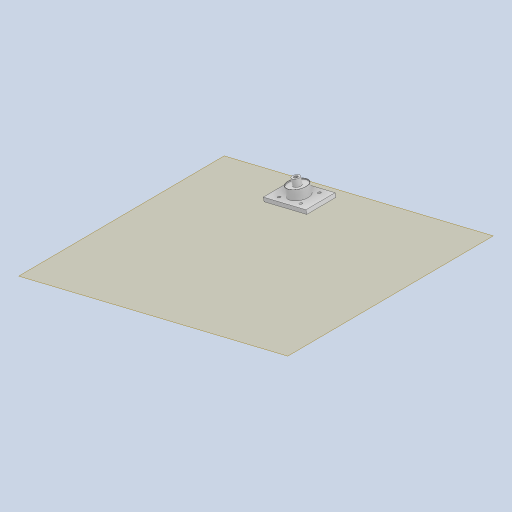
# Autodesk Inventor part: ступица
Saved by Autodesk Inventor 2024.2 (Build 282272000, 272)
## iProperties
Created: 2025-12-13
Part Number: ступица
Material: Типовые
Document SubType Name: Modeling
Designer: katya_notebook
Density: 1 g/cm^3
Appearance: По умолчанию
Author: katya_notebook
Autodesk Inventor part; units mm, degrees
ref_plane "РабПлоскость1" through (-284.2189, -273.5664, -69.8717) normal (-0.2311474, 0.9729175, 0.0015373) x (-0.972896, -0.2311526, 0.0064703)
sketch "Эскиз1" plane through (-284.2189, -273.5664, -69.8717) normal (-0.2311474, 0.9729175, 0.0015373) x (-0.972896, -0.2311526, 0.0064703)
  line L0 (22.5, -101.5) -> (54.25, -101.5)
  line L1 (54.25, -101.5) -> (54.25, -69.75)
  line L2 (54.25, -69.75) -> (22.5, -69.75)
  line L3 (22.5, -69.75) -> (22.5, -101.5)
  circle A0 centre (38.375, -85.625) radius 15.75 projected
  line L4 (38.375, -101.375) -> (38.375, -107.7067)
  point P0 (-339.2989, 71.7603)
  point P1 (22.5, -91.5)
  point P2 (38.375, -101.375)
  point P3 (38.375, -102.625)
  dimension "d0" = 31.75
  dimension "d1" = 31.75
  constraints: 10 end point, 2 parallel, 2 point on circle, 1 horizontal, 1 perpendicular, 1 point on line, 1 vertical, 1 other
  measures "d0" distance of L2.end L0.start
  measures "d1" distance of L1.end L2.end
extrude "Выдавливание1" add sketch "Эскиз1" along normal blind 4 contours L3 L2 L1 L0 | A0
sketch "Эскиз2" plane through (-285.1435, -269.6747, -69.8655) normal (-0.2311474, 0.9729175, 0.0015373) x (0.972896, 0.2311526, -0.0064703)
  line L0 (-54.25, 101.5) -> (-54.25, 69.75) projected
  line L1 (-54.25, 85.625) -> (-22.5, 85.625)
  line L2 (-22.5, 69.75) -> (-22.5, 101.5) projected
  line L3 (-54.25, 69.75) -> (-22.5, 69.75) projected
  line L4 (-50.375, 85.625) -> (-50.375, 101.5)
  line L5 (-36.5891, 93.625) -> (-22.5, 93.625)
  line L6 (-36.5891, 93.625) -> (-54.25, 93.625)
  line L7 (-50.375, 85.625) -> (-50.375, 68.9602)
  line L8 (-50.375, 75.625) -> (-22.5, 75.625)
  line L9 (-26.375, 103.5) -> (-26.375, 69.75)
  circle A0 centre (-50.375, 75.625) radius 2
  circle A1 centre (-26.375, 75.625) radius 2
  line L10 (-38.375, 72.7459) -> (-38.375, 103.5)
  line L11 (-38.375, 72.7459) -> (-38.375, 69.75)
  point P0 (339.2989, -71.7603)
  point P1 (-49.5, 101.5)
  point P2 (-38.375, 101.5)
  point P3 (-22.5, 85.625)
  point P4 (-54.25, 101.5)
  dimension "d5" = 8
  dimension "d6" = 12
  dimension "d7" = 10
  dimension "d8" = 4
  dimension "d9" = 4
  dimension "d16" = 12
  constraints: 18 end point, 7 point on line, 3 midpoint, 2 centre point, 2 horizontal, 2 perpendicular, 1 coincident, 1 vertical, 3 other
  measures "d5" distance of point (-22.5, 85.625) L5.end
  measures "d6" distance of L9.start L10.end
  measures "d7" distance of L4.start L8.start
  measures "d8" diameter of A1
  measures "d9" diameter of A0
  measures "d16" distance from line of L10 L8.start
sketch "Эскиз3" plane through (-285.1435, -269.6747, -69.8655) normal (-0.2311474, 0.9729175, 0.0015373) x (0.972896, 0.2311526, -0.0064703)
  circle A0 centre (-50.375, 95.625) radius 2
  circle A1 centre (-26.375, 95.625) radius 2
  line L0 (-54.25, 69.75) -> (-22.5, 69.75) projected
  line L1 (-38.375, 69.75) -> (-38.375, 101.5)
  line L2 (-38.375, 101.5) -> (-54.25, 85.625)
  line L3 (-54.25, 85.625) -> (-22.5, 85.625)
  point P0 (339.2989, -71.7603)
  point P1 (-50.375, 93.5625)
  dimension "d10" = 4
  dimension "d11" = 4
  dimension "d17" = 7.9375
  dimension "d18" = 15.875
  dimension "d19" = 10
  dimension "d20" = 10
  dimension "d21" = 12
  constraints: 6 end point, 2 centre point, 1 midpoint, 1 perpendicular
  measures "d10" diameter of A1
  measures "d11" diameter of A0
  measures "d17" distance from line of point (-50.375, 93.563) L3
  measures "d18" distance between parallel lines of L0 L3
  measures "d19" distance from line of L3 A0.centre
  measures "d20" distance from line of L3 A1.centre
  measures "d21" distance from line of L1 A1.centre
extrude "Выдавливание2" cut sketch "Эскиз3" against normal blind 10 contours A0 | A1
extrude "Выдавливание3" cut sketch "Эскиз2" against normal blind 10 contours A0 L8 L7 | L7 A0 | L7 L8 A0 | A1 L8 L9 | L9 L8 A1 | L8 L9 A1 | L9 L8 A1
sketch "Эскиз4" plane through (-285.1435, -269.6747, -69.8655) normal (-0.2311474, 0.9729175, 0.0015373) x (0.972896, 0.2311526, -0.0064703)
  line L0 (-54.25, 101.5) -> (-54.25, 69.75) projected
  line L1 (-54.25, 85.625) -> (-22.5, 85.625)
  line L2 (-22.5, 69.75) -> (-22.5, 101.5) projected
  line L3 (-38.375, 101.5) -> (-38.375, 69.75)
  line L4 (-54.25, 69.75) -> (-22.5, 69.75) projected
  circle A0 centre (-38.375, 85.625) radius 3.9
  point P0 (339.2989, -71.7603)
  dimension "d22" = 7.8
  constraints: 4 end point, 4 midpoint, 1 centre point
  measures "d22" diameter of A0
extrude "Выдавливание4" add sketch "Эскиз4" along normal blind 15.5 contours A0 L3 L1 | L1 L3 A0 | L3 A0 L1 | L1 A0 L3
sketch "Эскиз5" plane through (-326.6306, -263.465, -155.2165) normal (-0.2311474, 0.9729175, 0.0015373) x (0.9729187, 0.2311477, 0)
  circle A0 centre (0, 0) radius 2
  point P0 (378.6843, -154.9383)
  dimension "d25" = 4
  constraints: 1 centre point
  measures "d25" diameter of A0
extrude "Выдавливание5" cut sketch "Эскиз5" against normal blind 7
thread "Резьба1" size "M4x0.7" class "6H" standard "ANSI Metric M Profile" full length
sketch "Эскиз6" plane through (-337.6735, -286.1064, -171.0184) normal (-0.972896, -0.2311526, 0.0064703) x (0.0066504, 0, 0.9999779)
  line L0 (0, 4) -> (31.75, 4) projected
  line L1 (31.75, 4) -> (0, 4)
  line L2 (0, 4) -> (0, 0)
  line L3 (0, 0) -> (31.75, 0)
  line L4 (31.75, 0) -> (31.75, 4)
  point P0 (173.2603, 200.5685)
  point P1 (0, 4)
  constraints: 8 end point, 2 parallel, 1 horizontal, 1 perpendicular
ref_plane "РабПлоскость2" through (-345.4521, -286.2315, -166.64) normal (0.972896, 0.2311526, -0.0064703) x (-0.2311474, 0.9729175, 0.0015373)
extrude "Выдавливание6" add sketch "Эскиз6" along normal up to surface (7.625 mm away)
sketch "Эскиз7" plane through (-306.5729, -278.7673, -139.4745) normal (0.972896, 0.2311526, -0.0064703) x (-0.0066504, 0, -0.9999779)
  line L0 (0, 0) -> (31.75, 0) projected
  line L1 (0, 4) -> (31.75, 4) projected
  line L2 (31.75, 0) -> (0, 0)
  line L3 (0, 0) -> (0, 4)
  line L4 (0, 4) -> (31.75, 4)
  line L5 (31.75, 4) -> (31.75, 0)
  point P0 (-141.5103, 200.5685)
  point P1 (31.75, 4)
  constraints: 8 end point, 2 parallel, 1 horizontal, 1 perpendicular
ref_plane "РабПлоскость3" through (-299.726, -275.3674, -166.9441) normal (-0.972896, -0.2311526, 0.0064703) x (0.0066504, 0, 0.9999779)
extrude "Выдавливание7" add sketch "Эскиз7" along normal up to surface (7.625 mm away)
sketch "Эскиз8" plane through (-285.1435, -269.6747, -69.8655) normal (-0.2311474, 0.9729175, 0.0015373) x (0.972896, 0.2311526, -0.0064703)
  circle A0 centre (-38.375, 85.625) radius 3.9 projected
  circle A1 centre (-38.375, 85.625) radius 10
  point P0 (339.2989, -71.7603)
  dimension "d34" = 20
  constraints: 1 centre point, 1 coincident
  measures "d34" diameter of A1
extrude "Выдавливание8" add sketch "Эскиз8" along normal blind 8.5
sketch "Эскиз9" plane through (-285.1435, -269.6747, -69.8655) normal (-0.2311474, 0.9729175, 0.0015373) x (0.972896, 0.2311526, -0.0064703)
  circle A0 centre (-26.375, 75.625) radius 2 projected
  circle A1 centre (-26.375, 95.625) radius 2 projected
  circle A2 centre (-50.375, 75.625) radius 2 projected
  circle A3 centre (-50.375, 95.625) radius 2 projected
  circle A4 centre (-26.375, 75.625) radius 1.5
  circle A5 centre (-26.375, 95.625) radius 1.5
  circle A6 centre (-50.375, 95.625) radius 1.5
  circle A7 centre (-50.375, 75.625) radius 1.5
  point P0 (339.2989, -71.7603)
  dimension "d37" = 3
  dimension "d38" = 3
  dimension "d39" = 3
  dimension "d40" = 3
  constraints: 4 centre point, 4 coincident
  measures "d37" diameter of A4
  measures "d38" diameter of A7
  measures "d39" diameter of A6
  measures "d40" diameter of A5
ref_plane "РабПлоскость4" through (-375.5638, -295.1043, -173.6384) normal (-0.2311474, 0.9729175, 0.0015373) x (0.0066504, 0, 0.9999779)
extrude "Выдавливание9" add sketch "Эскиз9" against normal up to surface (4 mm away)
sketch "Эскиз10" plane through (-325.0126, -270.2754, -155.2273) normal (-0.2311474, 0.9729175, 0.0015373) x (0.9729187, 0.2311477, 0)
  circle A0 centre (0, 0) radius 9.75
  circle A1 centre (0, 0) radius 10
  point P0 (378.6843, -154.9383)
  dimension "d43" = 20
  dimension "d44" = 19.5
  constraints: 2 centre point, 1 coincident
  measures "d43" diameter of A1
  measures "d44" diameter of A0
extrude "Выдавливание10" add sketch "Эскиз10" along normal blind 1
